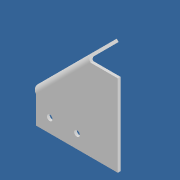
# Autodesk Inventor part: CoreXY_Angle
Saved by Autodesk Inventor 2020 (Build 240168000, 168)
## iProperties
Created: 2021-05-05
Part Number: CoreXY_Angle
Material: 一般
Document SubType Name: Sheet Metal
Designer: ken113
Density: 1 g/cm^3
Sheet Metal Rule: Default_mm
Appearance: 既定
Author: ken113
Autodesk Inventor part; units mm, degrees
ref_plane "YZ Plane" through (0, 0, 0) normal (1, 0, 0) x (0, 1, 0)
ref_plane "XZ Plane" through (0, 0, 0) normal (0, 1, 0) x (-1, 0, 0)
ref_plane "XY Plane" through (0, 0, 0) normal (0, 0, 1) x (1, 0, 0)
sketch "スケッチ1" plane through (0, 0, 0) normal (0, 0, 1) x (1, 0, 0)
  line L0 (0, 0) -> (80, 80)
  line L1 (80, 80) -> (80, 0)
  line L2 (80, 0) -> (0, 0)
  dimension "d0" = 45
  dimension "d1" = 80
  measures "d0" angle of L0 L2
  measures "d1" distance of L1.end L0.start
extrude "プレート1" add sketch "スケッチ1" along normal blind 2
sketch "スケッチ2" plane through (0, 0, 2) normal (0, 0, 1) x (1, 0, 0)
  line L0 (0, 0) -> (80, 80) projected
  line L1 (0, 0) -> (20, 0)
  line L2 (20, 0) -> (20, 20)
  line L3 (20, 20) -> (0, 20)
  line L4 (0, 20) -> (0, 0)
  line L5 (80, 80) -> (60, 80)
  line L6 (60, 80) -> (60, 60)
  line L7 (60, 60) -> (80, 60)
  line L8 (80, 60) -> (80, 80)
  line L9 (0, 0) -> (80, 80) projected
  dimension "d3" = 20
  dimension "d6" = 20
  constraints: 16 end point, 4 parallel, 2 horizontal, 2 perpendicular, 2 point on line
  measures "d3" distance of L2.end L3.end
  measures "d6" distance of L5.end L6.end
extrude "押し出し1" cut sketch "スケッチ2" against normal blind 10 contours L0 L2 L1 | L6 L5 L0 | L0 L8 L7
sketch "スケッチ3" plane through (0, 0, 2) normal (0, 0, 1) x (1, 0, 0)
  line L0 (20, 20) -> (20, 0) projected
  line L1 (80, 0) -> (20, 0) projected
  line L2 (80, 60) -> (80, 0) projected
  line L3 (80, 60) -> (60, 60) projected
  line L4 (20, 20) -> (60, 60) projected
  line L5 (20, 20) -> (60, 60) projected
  line L6 (20, 20) -> (18.5858, 21.4142)
  line L7 (18.5858, 21.4142) -> (58.5858, 61.4142)
  line L8 (58.5858, 61.4142) -> (60, 60)
  point P0 (0, 0)
  dimension "d7" = 2
  constraints: 6 end point, 3 perpendicular
  measures "d7" distance of L0.start L6.end
extrude "押し出し2" add sketch "スケッチ3" against normal up to surface (2 mm away) contours L6 L7 L8 L4
sketch "スケッチ4" plane through (58.5858, 61.4142, 0) normal (-0.7071068, 0.7071068, 0) x (-0.7071068, -0.7071068, 0)
  line L0 (56.5685, 0) -> (0, 0)
  line L1 (0, 0) -> (0, -20)
  line L2 (0, -20) -> (56.5685, -20)
  line L3 (56.5685, -20) -> (56.5685, 0)
  constraints: 6 end point, 1 horizontal, 1 perpendicular, 1 vertical
edge flange "フランジ1" height 22 angle 90 thickness 2 bend radius 2 thickness toward (-0.7071068, 0.7071068, 0) relief tear relief width 2 relief depth 1 edges at (38.5858, 41.4142, 0) wall of the first edge with corners at (18.5858, 21.4142, 0) (58.5858, 61.4142, 0) (58.5858, 61.4142, -20) (18.5858, 21.4142, -20)
bend "曲げ1"
corner "コーナー1"
sketch "スケッチ5" plane through (18.5858, 21.4142, -2) normal (0.7071068, -0.7071068, 0) x (-0.7071068, -0.7071068, 0)
  line L0 (-56.5685, 0) -> (0, 0) projected
  line L1 (0, 0) -> (0, 18) projected
  line L2 (0, 18) -> (-56.5685, 18) projected
  line L3 (-56.5685, 0) -> (-56.5685, 18) projected
  line L4 (-56.5685, 0) -> (0, 0) projected
  point P0 (28.2843, -2)
  point P1 (-50.7843, 8)
  point P2 (-5.7843, 8)
  point P3 (-28.2843, 8)
  point P4 (-28.2843, 0)
  point P5 (-28.2843, 0)
  dimension "d20" = 10
  dimension "d23" = 45
  dimension "d24" = 22.5
  constraints: 2 horizontal alignment, 2 midpoint, 1 vertical alignment
  measures "d20" distance from line of point (-50.784, 8) L2
  measures "d23" distance of point (-50.784, 8) point (-5.784, 8)
  measures "d24" distance of point (-50.784, 8) point (-28.284, 8)
hole "穴1" at (54.4957, 57.3241, -10) at (22.6759, 25.5043, -10) at (38.5858, 41.4142, -10) direction (-0.7071068, 0.7071068, 0) diameter 4.2 depth 2
sketch "スケッチ6" plane through (0, 0, 2) normal (0, 0, 1) x (1, 0, 0)
  line L0 (80, 0) -> (20, 0) projected
  line L1 (20, 20) -> (20, 0) projected
  line L2 (80, 60) -> (80, 0) projected
  point P0 (0, 0)
  point P1 (30, 10)
  point P2 (70, 10)
  point P3 (50, 10)
  dimension "d32" = 10
  dimension "d33" = 10
  dimension "d34" = 10
  dimension "d35" = 20
  measures "d32" distance from line of point (30, 10) L0
  measures "d33" distance from line of point (30, 10) L1
  measures "d34" distance from line of L2 point (70, 10)
  measures "d35" distance of point (30, 10) point (50, 10)
hole "穴2" at (30, 10, 2) at (50, 10, 2) direction (0, 0, -1) diameter 4.2 depth 2
equation "\"d24\" = 0.5 * d23"
equation "\"d30\" = Thickness"
equation "\"d41\" = Thickness"
equation "\"d2\" = Thickness"
equation "\"d10\" = BendReliefWidth"
equation "\"d11\" = BendReliefDepth"
equation "\"d12\" = MinimumRemnant"
equation "\"d13\" = TransitionRadius"
equation "\"d16\" = BendRadius"
equation "\"d17\" = CornerReliefSize"
equation "\"d18\" = GapSize"
equation "\"d19\" = JacobiRadiusSize"
equation "\"BendRadius\" = Thickness"
equation "\"BendReliefWidth\" = Thickness"
equation "\"BendReliefDepth\" = 0.5 * Thickness"
equation "\"CornerReliefSize\" = 4 * Thickness"
equation "\"MinimumRemnant\" = 2 * Thickness"
equation "\"TransitionRadius\" = BendRadius"
equation "\"JacobiRadiusSize\" = BendRadius"
equation "\"GapSize\" = Thickness"
equation "\"Thickness\" = 2"
